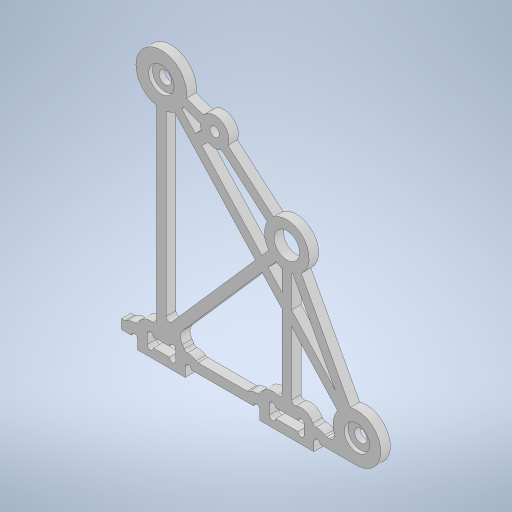
# Autodesk Inventor part: 左フレーム
Saved by Autodesk Inventor 2023 (Build 270158000, 158)
## iProperties
Created: 2022-06-19
Part Number: 左フレーム
Material: 一般
Document SubType Name: Modeling
Designer: muzho
Density: 1 g/cm^3
Appearance: 既定
Author: muzho
Autodesk Inventor part; units mm, degrees
ref_plane "YZ Plane" through (0, 0, 0) normal (1, 0, 0) x (0, 1, 0)
ref_plane "XZ Plane" through (0, 0, 0) normal (0, 1, 0) x (-1, 0, 0)
ref_plane "XY Plane" through (0, 0, 0) normal (0, 0, 1) x (1, 0, 0)
sketch "スケッチ1" plane through (0, 0, 0) normal (0, 0, 1) x (1, 0, 0)
  circle A0 centre (52, 42.9528) radius 4.025
  circle A1 centre (29.2913, 62.5568) radius 1.5
  circle A2 centre (74.0428, 1.5165) radius 4
  circle A3 centre (12.5499, 68.38) radius 4
  circle A4 centre (12.5499, 68.38) radius 8
  circle A5 centre (29.2913, 62.5568) radius 4.5
  circle A6 centre (52, 42.9528) radius 7.025
  circle A7 centre (74.0428, 1.5165) radius 2
  circle A8 centre (74.0428, 1.5165) radius 7.5165
  line L0 (12.5499, 68.38) -> (29.2913, 62.5568) construction
  line L1 (20.4646, 67.2151) -> (25.7769, 65.3673)
  line L2 (24.7914, 62.5338) -> (19.4791, 64.3816)
  line L3 (29.2913, 62.5568) -> (52, 42.9528) construction
  line L4 (31.5226, 58.6489) -> (45.8248, 46.3021)
  line L5 (33.483, 60.9198) -> (47.7852, 48.573)
  line L6 (12.5499, 68.38) -> (74.0428, 1.5165) construction
  line L7 (16.7652, 61.5806) -> (67.9529, 5.9223)
  line L8 (18.9733, 63.6114) -> (67.2164, 11.155)
  line L9 (29.2913, 62.5568) -> (24.2268, 57.8991) construction
  line L10 (25.1531, 60.7889) -> (23.2114, 59.0031)
  line L11 (27.1839, 58.5807) -> (25.2422, 56.795)
  line L12 (-37.0636, -3) -> (111.1776, -3) construction
  line L13 (12.5499, 68.38) -> (12.5499, -15.8691) construction
  circle A9 centre (9.0499, -3) radius 1
  circle A10 centre (9.0499, -6) radius 1
  circle A11 centre (4.0499, -6) radius 1
  line L14 (8.0499, -6) -> (5.0499, -6)
  line L15 (8.0499, -3) -> (8.0499, -6)
  line L16 (5.0499, -6) -> (5.0499, -9)
  line L17 (5.0499, -9) -> (12.5499, -9)
  line L18 (3.0499, -6) -> (0.0499, -6)
  line L19 (0.0499, -6) -> (0.0499, -3)
  circle A12 centre (16.0499, -6) radius 1
  circle A13 centre (16.0499, -3) radius 1
  line L20 (17.0499, -3) -> (17.0499, -6)
  line L21 (17.0499, -6) -> (20.0499, -6)
  line L22 (20.0499, -9) -> (12.5499, -9)
  line L23 (20.0499, -6) -> (20.0499, -9)
  circle A14 centre (21.0499, -6) radius 1
  line L24 (22.0499, -6) -> (25.0499, -6)
  line L25 (25.0499, -6) -> (25.0499, -3)
  line L26 (10.0499, -3) -> (12.5499, -3)
  line L27 (10.0499, -6) -> (12.5499, -6)
  line L28 (15.0499, -3) -> (12.5499, -3)
  line L29 (15.0499, -6) -> (12.5499, -6)
  arc A15 (1.0499, -3) -> (1.6499, -2.8) centre (1.0499, -2) ccw
  arc A16 (4.378, -2.0135) -> (1.6499, -2.8) centre (4.0499, -6) ccw
  line L30 (1.0499, -3) -> (0.0499, -3)
  arc A17 (4.378, -2.0135) -> (5.378, -1.4135) centre (4.46, -1.0168) ccw
  arc A18 (9.8499, 0.9192) -> (5.378, -1.4135) centre (9.0499, -3) ccw
  arc A19 (9.8499, 0.9192) -> (11.0499, 1.899) centre (10.0499, 1.899) ccw
  line L31 (24.0499, -3) -> (25.0499, -3)
  arc A20 (23.4499, -2.8) -> (24.0499, -3) centre (24.0499, -2) ccw
  arc A21 (23.4499, -2.8) -> (20.7218, -2.0135) centre (21.0499, -6) ccw
  line L32 (52, 42.9528) -> (9.0499, -6) construction
  line L33 (48.6013, 36.8047) -> (19.2558, 3.3578)
  line L34 (15.8016, 3.9697) -> (46.3462, 38.7832)
  arc A22 (19.7218, -1.4135) -> (19.1704, -0.4975) centre (16.0499, -3) ccw
  arc A23 (19.7218, -1.4135) -> (20.7218, -2.0135) centre (20.6398, -1.0168) ccw
  arc A24 (19.2558, 3.3578) -> (19.1704, -0.4975) centre (21.5108, 1.3793) ccw
  line L35 (11.0499, 1.899) -> (11.0499, 60.5218)
  line L36 (14.0499, 60.5218) -> (14.0499, 4.6292)
  arc A25 (14.0499, 4.6292) -> (15.8016, 3.9697) centre (15.0499, 4.6292) ccw
  line L37 (52, 42.9528) -> (52, -12.1478) construction
  circle A26 centre (47.5, -3) radius 1
  circle A27 centre (47.5, -6) radius 1
  line L38 (46.5, -3) -> (46.5, -6)
  line L39 (48.5, -3) -> (52, -3)
  line L40 (48.5, -6) -> (52, -6)
  circle A28 centre (42.5, -6) radius 1
  line L41 (46.5, -6) -> (43.5, -6)
  line L42 (41.5, -6) -> (38.5, -6)
  line L43 (38.5, -6) -> (38.5, -3)
  line L44 (39.5, -3) -> (38.5, -3)
  arc A29 (39.5, -3) -> (40.1, -2.8) centre (39.5, -2) ccw
  arc A30 (42.8281, -2.0135) -> (40.1, -2.8) centre (42.5, -6) ccw
  arc A31 (42.8281, -2.0135) -> (43.8281, -1.4135) centre (42.9101, -1.0168) ccw
  arc A32 (49.1, 0.6661) -> (43.8281, -1.4135) centre (47.5, -3) ccw
  arc A33 (49.1, 0.6661) -> (50.5, 1.5826) centre (49.5, 1.5826) ccw
  line L45 (50.5, 36.0898) -> (50.5, 1.5826)
  line L46 (53.5, 36.0898) -> (53.5, 1.5826)
  arc A34 (60.1719, -1.4135) -> (54.9, 0.6661) centre (56.5, -3) ccw
  arc A35 (60.1719, -1.4135) -> (61.1719, -2.0135) centre (61.0899, -1.0168) ccw
  arc A36 (63.9, -2.8) -> (61.1719, -2.0135) centre (61.5, -6) ccw
  arc A37 (63.9, -2.8) -> (64.5, -3) centre (64.5, -2) ccw
  line L47 (64.5, -3) -> (65.5, -3)
  line L48 (65.5, -6) -> (65.5, -3)
  line L49 (62.5, -6) -> (65.5, -6)
  circle A38 centre (61.5, -6) radius 1
  line L50 (57.5, -6) -> (60.5, -6)
  line L51 (57.5, -3) -> (57.5, -6)
  circle A39 centre (56.5, -3) radius 1
  circle A40 centre (56.5, -6) radius 1
  line L52 (55.5, -6) -> (52, -6)
  line L53 (55.5, -3) -> (52, -3)
  line L54 (43.5, -6) -> (43.5, -9)
  line L55 (43.5, -9) -> (52, -9)
  line L56 (60.5, -9) -> (52, -9)
  line L57 (60.5, -6) -> (60.5, -9)
  line L58 (25.0499, -3) -> (38.5, -3)
  line L59 (25.0499, -6) -> (38.5, -6)
  line L60 (65.5, -6) -> (74.0428, -6)
  arc A41 (65.5, -3) -> (66.9467, -0.9622) centre (65.5, -1.4675) ccw
  line L61 (52, 42.9528) -> (74.0428, 1.5165) construction
  line L62 (56.5475, 37.5983) -> (71.908, 8.7234)
  line L63 (53.8989, 36.1893) -> (67.2164, 11.155)
  line L64 (67.2164, 11.155) -> (69.2581, 7.3169) construction
  line L65 (67.2164, 11.155) -> (70.1611, 7.9531) construction
  arc A42 (53.5, 1.5826) -> (54.9, 0.6661) centre (54.5, 1.5826) ccw
  circle A43 centre (12.5499, 68.38) radius 2
  point P0 (53.5, 21.6375)
  point P1 (42.1402, 33.9894)
  point P2 (50.5, 29.3313)
  point P3 (46.1726, 34.0366)
  point P4 (53.5, 26.0693)
  point P5 (44.1827, 31.7686)
  point P6 (50.5, 24.8995)
  point P7 (44.1302, 36.2575)
  dimension "d2" = 14.05
  dimension "d0" = 16
  dimension "d1" = 9
  dimension "d3" = 4
  dimension "d4" = 3
  dimension "d5" = 1.5
  dimension "d6" = 3
  dimension "d7" = 1.5
  dimension "d8" = 3
  dimension "d9" = 1.5
  dimension "d10" = 3
  dimension "d11" = 1.5
  dimension "d12" = 2
  dimension "d13" = 3.5
  dimension "d14" = 2
  dimension "d15" = 3
  dimension "d16" = 2
  dimension "d17" = 5
  dimension "d18" = 3
  dimension "d19" = 3
  dimension "d20" = 3
  dimension "d21" = 3
  dimension "d22" = 3
  dimension "d23" = 1
  dimension "d24" = 3
  dimension "d25" = 1
  dimension "d26" = 1
  dimension "d27" = 3
  dimension "d28" = 1.5
  dimension "d29" = 3
  dimension "d30" = 1
  dimension "d31" = 3
  dimension "d32" = 3
  dimension "d33" = 1.5
  dimension "d34" = 1
  dimension "d35" = 2
  dimension "d36" = 2
  dimension "d37" = 3
  dimension "d38" = 3
  dimension "d39" = 3.5
  dimension "d40" = 2
  dimension "d41" = 5
  dimension "d42" = 3
  dimension "d43" = 1
  dimension "d44" = 1
  dimension "d45" = 1
  dimension "d46" = 3
  dimension "d47" = 3
  dimension "d48" = 3
  dimension "d49" = 1.5
  dimension "d50" = 3
  dimension "d51" = 3
  dimension "d52" = 1.5
  dimension "d55" = 4
  constraints: 130 end point, 81 point on circle, 41 centre point, 38 symmetric about line, 22 tangent, 17 parallel, 9 point on line, 8 horizontal, 8 perpendicular, 8 vertical, 6 coincident, 5 horizontal alignment, 4 concentric, 1 vertical alignment, 47 other
  measures "d0" diameter of A4
  measures "d1" diameter of A5
  measures "d3" diameter of A7
  measures "d4" distance between parallel lines of L2 L1
  measures "d5" distance between parallel lines of L2 L0
  measures "d6" distance between parallel lines of L4 L5
  measures "d7" distance between parallel lines of L4 L3
  measures "d8" distance between parallel lines of L7 L8
  measures "d9" distance between parallel lines of L7 L6
  measures "d10" distance between parallel lines of L11 L10
  measures "d11" distance between parallel lines of L10 L9
  measures "d12" diameter of A9
  measures "d13" distance from line of L13 A9.centre
  measures "d14" diameter of A10
  measures "d15" distance of L32.end A9.centre
  measures "d16" diameter of A11
  measures "d17" distance of L32.end A11.centre
  measures "d18" length of L14
  measures "d19" distance of L14.end L16.end
  measures "d20" distance of L18.start L18.end
  measures "d21" distance of L18.end L19.end
  measures "d22" radial gap between concentric circles of A9 A18
  measures "d23" radius of A17
  measures "d24" radial gap between concentric circles of A11 A16
  measures "d25" radius of A15
  measures "d26" radius of A19
  measures "d27" distance between parallel lines of L33 L34
  measures "d28" distance between parallel lines of L33 L32
  measures "d30" radius of A23
  measures "d31" radius of A24
  measures "d32" distance between parallel lines of L35 L36
  measures "d33" distance between parallel lines of L35 L13
  measures "d34" radius of A25
  measures "d35" diameter of A26
  measures "d36" diameter of A27
  measures "d37" distance of L38.start L38.end
  measures "d38" distance between parallel lines of L40 L39
  measures "d39" distance of L40.start L40.end
  measures "d40" diameter of A28
  measures "d41" distance of A27.centre A28.centre
  measures "d42" distance of L42.start L42.end
  measures "d43" radius of A31
  measures "d44" radius of A29
  measures "d45" radius of A33
  measures "d46" radial gap between concentric circles of A28 A30
  measures "d47" radial gap between concentric circles of A26 A32
  measures "d48" distance between parallel lines of L45 L46
  measures "d49" distance between parallel lines of L45 L37
  measures "d50" distance of L41.end L54.end
  measures "d51" distance between parallel lines of L63 L62
  measures "d52" distance between parallel lines of L63 L61
  measures "d55" diameter of A43
extrude "押し出し1" add sketch "スケッチ1" along normal blind 3 contours A4 | A4 L36 A25 L34 L7 L33 A24 A22 A23 A21 A20 L31 L25 L24 A14 L21 L20 A13 L28 L26 A9 L15 L14 A11 L18 L19 L30 A15 A16 A17 A18 A19 L35 | L1 A5 L2 A4 | A5 | A4 L8 L34 L7 | L34 L8 L33 L7 | L10 A5 L11 L8 | L5 A6 L4 A5 | L33 L8 L45 L7 | L34 A6 L33 L8 | A6 | L45 L8 L46 L7 | L7 L46 A42 A34 A35 A36 A37 L47 L48 L49 A38 L50 L51 A39 L53 L39 A26 L38 L41 A28 L42 L43 L44 A29 A30 A31 A32 A33 L45 | L46 L8 L63 A6 L62 A8 L7 | L45 A6 L46 L8 | A8 | A8 L60 L48 A41 | L14 A10 L27 L29 A12 L21 L23 L22 L17 L16 | L58 L43 L59 L25 | L57 L56 L55 L54 L41 A27 L40 L52 A40 L50
extrude "押し出し2" add sketch "スケッチ1" along normal blind 1.8 contours A2 | A3
equation "\"d5\" = 0.5 * d4"
equation "\"d7\" = 0.5 * d6"
equation "\"d9\" = 0.5 * d8"
equation "\"d11\" = 0.5 * d10"
equation "\"d28\" = 0.5 * d27"
equation "\"d33\" = 0.5 * d32"
equation "\"d49\" = 0.5 * d48"
equation "\"d52\" = 0.5 * d51"
